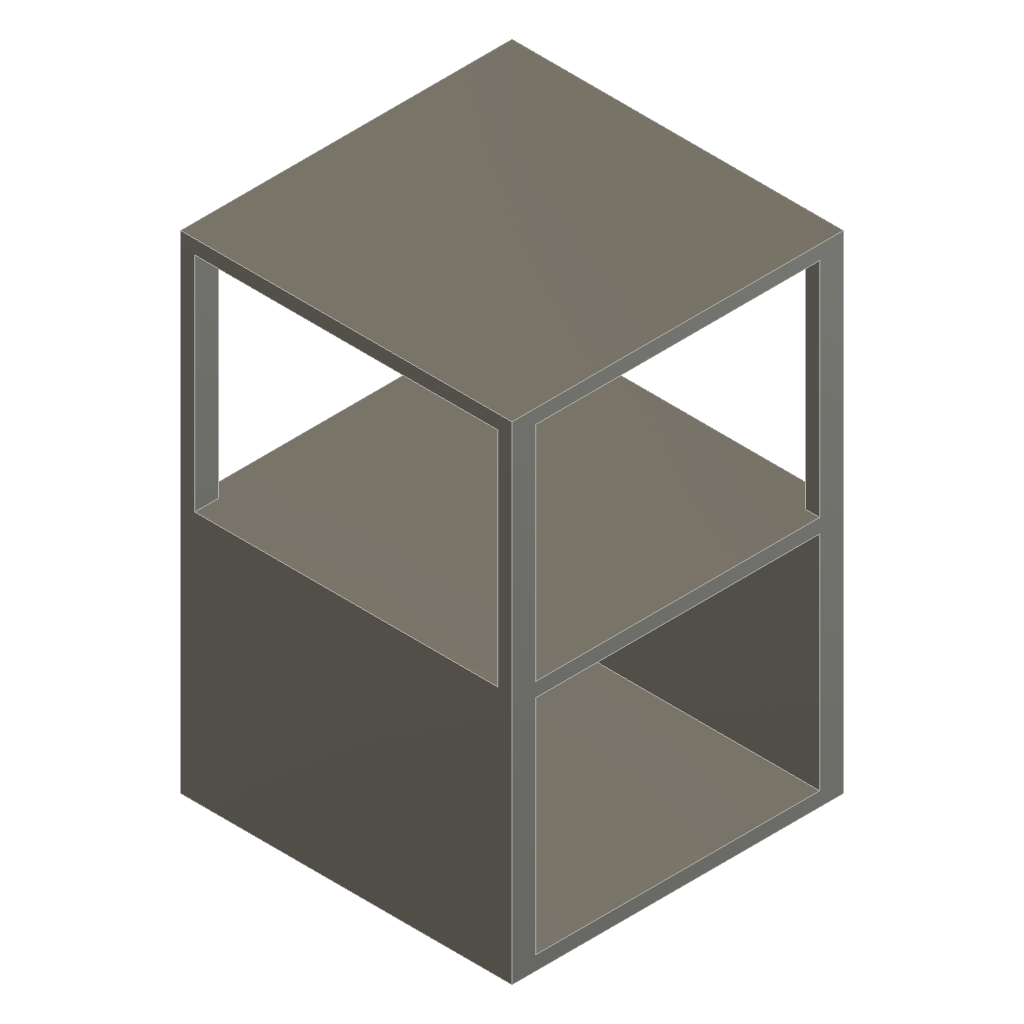
SelfBalBot-f3d (Autodesk Fusion 360 design; units mm, degrees)
part number: 2026-10-06-11-52-30-977
Autodesk Fusion 360 part; units mm, degrees
sketch "Sketch1" plane through (0, 0, 0) normal (0, 1, 0) x (1, 0, 0)
  line L0 (-25, 30) -> (45, 30)
  line L1 (45, 30) -> (45, -40)
  line L2 (45, -40) -> (-25, -40)
  line L3 (-25, -40) -> (-25, 30)
  dimension "d1" = 70
  dimension "d2" = 70
  constraint horizontal L0
  constraint vertical L1
  constraint horizontal L2
  constraint vertical L3
  measures "d1" distance of L0.start L0.end
  measures "d2" distance of L0.start L2.end
extrude "Extrude1" add sketch "Sketch1" against normal blind 3
sketch "Sketch2" plane through (0, 0, 0) normal (0, 1, 0) x (-1, 0, 0)
  line L0 (25, 40) -> (-45, 40)
  line L1 (-45, 40) -> (-45, -30)
  line L2 (-45, -30) -> (25, -30)
  line L3 (25, -30) -> (25, 40)
  line L4 (25, 35) -> (-45, 35)
  line L5 (-45, 35) -> (-45, 40)
  line L6 (-45, 40) -> (25, 40)
  line L7 (25, 40) -> (25, 35)
  constraint horizontal L4
  constraint vertical L5
  constraint horizontal L6
  constraint vertical L7
  constraint coincident L0.end L1.start
  constraint coincident L3 L4.start
sketch "Sketch3" plane through (0, 0, 0) normal (0, 1, 0) x (-1, 0, 0)
  line L0 (25, -30) -> (-45, -30)
  line L1 (-45, -30) -> (-45, -25)
  line L2 (-45, -25) -> (25, -25)
  line L3 (25, -25) -> (25, -30)
  constraint horizontal L0
  constraint vertical L1
  constraint horizontal L2
  constraint vertical L3
extrude "Extrude2" add sketch "Sketch2" sketch "Sketch3" along normal blind 50 contours L0 L1 L3 L4 L5 L6 L7 of sketch 2
sketch "Sketch4" plane through (0, 0, -25) normal (0, 0, 1) x (1, 0, 0)
  line L0 (-25, 0) -> (45, 0)
  line L1 (45, 0) -> (45, 50)
  line L2 (45, 50) -> (-25, 50)
  line L3 (-25, 50) -> (-25, 0)
  line L4 (-25, 50) -> (45, 50)
  line L5 (45, 50) -> (45, 47)
  line L6 (45, 47) -> (-25, 47)
  line L7 (-25, 47) -> (-25, 50)
  constraint horizontal L4
  constraint vertical L5
  constraint horizontal L6
  constraint vertical L7
  constraint coincident L1 L5.end
  constraint coincident L2.end L3.start
extrude "Extrude3" add sketch "Sketch4" along normal blind 60 contours L1 L2 L3 L4 L5 L6 L7
sketch "Sketch5" plane through (0, 50, 0) normal (0, 1, 0) x (-1, 0, 0)
  line L0 (-45, 40) -> (-45, -30)
  line L1 (-45, -30) -> (25, -30)
  line L2 (25, -30) -> (25, 40)
  line L3 (25, 40) -> (-45, 40)
  line L4 (25, 40) -> (22, 40)
  line L5 (22, 40) -> (22, -30)
  line L6 (22, -30) -> (25, -30)
  line L7 (25, -30) -> (25, 40)
  dimension "d9" = 3
  constraint horizontal L4
  constraint vertical L5
  constraint horizontal L6
  constraint vertical L7
  constraint coincident L2.end L3.start
  measures "d9" distance of L2.end L4.end
sketch "Sketch6" plane through (0, 50, 0) normal (0, 1, 0) x (-1, 0, 0)
  line L0 (-45, 40) -> (-42, 40)
  line L1 (-42, 40) -> (-42, -30)
  line L2 (-42, -30) -> (-45, -30)
  line L3 (-45, -30) -> (-45, 40)
  dimension "d10" = 3
  constraint horizontal L0
  constraint vertical L1
  constraint horizontal L2
  constraint vertical L3
  measures "d10" distance of L0.start L0.end
extrude "Extrude4" add sketch "Sketch6" sketch "Sketch5" along normal blind 50 of sketch 2 contours L1 L2 L3 L4 L5 L6 L7
sketch "Sketch7" plane through (-22, 0, 0) normal (1, 0, 0) x (0, 0, -1)
  line L0 (-40, 50) -> (30, 50)
  line L1 (30, 50) -> (30, 100)
  line L2 (30, 100) -> (-40, 100)
  line L3 (-40, 100) -> (-40, 50)
  line L4 (-40, 100) -> (30, 100)
  line L5 (30, 100) -> (30, 97)
  line L6 (30, 97) -> (-40, 97)
  line L7 (-40, 97) -> (-40, 100)
  dimension "d13" = 3
  constraint horizontal L4
  constraint vertical L5
  constraint horizontal L6
  constraint vertical L7
  constraint coincident L2.end L3.start
  measures "d13" distance of L2.end L6.end
extrude "Extrude5" add sketch "Sketch7" along normal blind 64 contours L1 L2 L3 L4 L5 L6 L7
sketch "Sketch8" plane through (-25, 0, 0) normal (-1, 0, 0) x (0, 0, 1)
  line L0 (-30, 100) -> (-30, -3)
  line L1 (-30, -3) -> (40, -3)
  line L2 (40, -3) -> (40, 100)
  line L3 (40, 100) -> (-30, 100)
  line L4 (-25, 47) -> (35, 47)
  line L5 (35, 47) -> (35, 0)
  line L6 (35, 0) -> (-25, 0)
  line L7 (-25, 0) -> (-25, 47)
  line L8 (-25, 50) -> (35, 50)
  line L9 (35, 50) -> (35, 97)
  line L10 (35, 97) -> (-25, 97)
  line L11 (-25, 97) -> (-25, 50)
  dimension "d16" = 60
  dimension "d17" = 47
  constraint horizontal L8
  constraint vertical L9
  constraint horizontal L10
  constraint vertical L11
  measures "d16" distance of L8.start L8.end
  measures "d17" distance of L8.start L10.end
extrude "Extrude6" cut sketch "Sketch8" against normal blind 80 contours L8 L9 L10 L11
